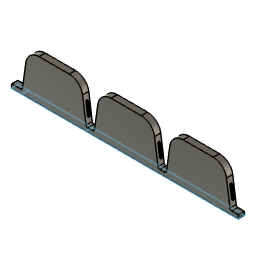
Drawer Organizer v13 (Autodesk Fusion 360 design; units mm, degrees)
Autodesk Fusion 360 part; units mm, degrees
sketch "Schizzo1" plane through (0, 0, 0) normal (0, 0, 1) x (1, 0, 0)
  line L0 (-97, 20) -> (158, 20)
  line L1 (158, 20) -> (158, 13)
  line L2 (158, 13) -> (-97, 13)
  line L3 (-97, 13) -> (-97, 20)
  line L4 (-85, 20) -> (-85, 13)
  line L5 (-13, 20) -> (-13, 13)
  dimension "d1" = 255
  dimension "d2" = 7
  dimension "d3" = 12
  dimension "d4" = 72
  constraint horizontal L0
  constraint vertical L1
  constraint horizontal L2
  constraint vertical L3
  constraint coincident L0 L4.start
  constraint coincident L2 L4.end
  constraint perpendicular L2 L4
  constraint coincident L0 L5.start
  constraint coincident L2 L5.end
  constraint perpendicular L2 L5
  measures "d1" distance of L0.start L0.end
  measures "d2" distance of L0.start L2.end
  measures "d3" distance of L3 L4
  measures "d4" distance of L4 L5
extrude "Estrusione1" add sketch "Schizzo1" along normal blind 4
extrude "Estrusione2" add sketch "Schizzo1" along normal blind 46 contours L0 L2 L4 L5
sketch "Schizzo2" plane through (0, 13, 0) normal (0, -1, 0) x (1, 0, 0)
  line L0 (-85, 4) -> (-97, 4)
  line L1 (-97, 4) -> (-97, 0)
  line L2 (-97, 0) -> (158, 0)
  line L3 (158, 0) -> (158, 4)
  line L4 (158, 4) -> (-13, 4)
  line L5 (-13, 4) -> (-13, 46)
  line L6 (-13, 46) -> (-85, 46)
  line L7 (-85, 46) -> (-85, 4)
  line L8 (-85, 46) -> (-13, 46) construction
  line L9 (-13, 46) -> (-13, 4) construction
  line L10 (-13, 4) -> (-85, 4) construction
  line L11 (-85, 4) -> (-85, 46) construction
  circle A0 centre (-66, 31) radius 15
  line L12 (-49, 46) -> (-49, 4) construction
  circle A1 centre (-32, 31) radius 15
  line L13 (-66, 46) -> (-32, 46)
  line L14 (-85, 4) -> (-80.8499, 33.1166)
  line L15 (-13, 4) -> (-17.1501, 33.1166)
  line L16 (-85, 4) -> (-13, 4)
  line L17 (-66, 46) -> (-85, 46)
  line L18 (-85, 46) -> (-85, 4)
  line L19 (-32, 46) -> (-13, 46)
  line L20 (-13, 46) -> (-13, 4)
  dimension "d9" = 15
  dimension "d10" = 34
  constraint horizontal L8
  constraint vertical L9
  constraint horizontal L10
  constraint vertical L11
  constraint coincident L4.end L5.start
  constraint coincident L6.end L7.start
  constraint tangent L8 A0
  constraint midpoint L8 L12.start
  constraint midpoint L10 L12.end
  constraint symmetric A0 L12 A1
  constraint coincident A0 L13.start
  constraint coincident A1 L13.end
  constraint coincident L8 L13.end
  constraint tangent A1 L13
  constraint coincident L0.start L7.end
  constraint coincident A0 L14.end
  constraint tangent A0 L14
  constraint symmetric L12 L0.start L4.end
  constraint symmetric L12 L14.end L15.end
  constraint perpendicular L11 L17
  constraint symmetric L6.end L12 L5.end
  constraint symmetric L12 L13.start L13.end
  measures "d9" radius of A0
  measures "d10" distance of A0.centre A1.centre
extrude "Estrusione3" cut sketch "Schizzo2" against normal blind 10 contours L6 L7 A0 L14 L17 L18 | L5 L6 A1 L15 L19 L20
pattern_linear "Serie R1" count 3 spacing 81 along (1, 0, 0) of "Estrusione2"
pattern_linear "Serie R2" count 3 spacing 81 along (1, 0, 0) of "Estrusione3"
sketch "Schizzo3" plane through (-83.8663, 0, 11.9537) normal (-0.989994, 0, 0.141107) x (0, -1, 0)
  line L0 (-20, 21.3768) -> (-20, -8.0341)
  line L1 (-20, -8.0341) -> (-13, -8.0341)
  line L2 (-13, -8.0341) -> (-13, 21.3768)
  line L3 (-13, 21.3768) -> (-20, 21.3768)
  line L4 (-20, 21.3768) -> (-13, 21.3768) construction
  line L5 (-13, 21.3768) -> (-13, -8.0341) construction
  line L6 (-13, -8.0341) -> (-20, -8.0341) construction
  line L7 (-20, -8.0341) -> (-20, 21.3768) construction
  line L8 (-16.5, 21.3768) -> (-16.5, -8.0341) construction
  line L9 (-15.8, -0.0341) -> (-17.2, -0.0341)
  line L10 (-17.2, -0.0341) -> (-17.2, 14.9659)
  line L11 (-17.2, 14.9659) -> (-15.8, 14.9659)
  line L12 (-15.8, 14.9659) -> (-15.8, -0.0341)
  line L13 (-15.8, -0.0341) -> (-17.2, 14.9659) construction
  line L14 (-17.2, -0.0341) -> (-15.8, 14.9659) construction
  point P0 (-16.5, 7.4659)
  dimension "d21" = 1.4
  dimension "d22" = 15
  dimension "d23" = 8
  constraint horizontal L4
  constraint vertical L5
  constraint horizontal L6
  constraint vertical L7
  constraint coincident L0.start L3.end
  constraint coincident L1.end L2.start
  constraint midpoint L4 L8.start
  constraint midpoint L6 L8.end
  constraint horizontal L9
  constraint perpendicular L9 L10
  constraint parallel L9 L11
  constraint parallel L10 L12
  constraint coincident L13 P0
  constraint coincident L14 P0
  constraint coincident L8 P0
  measures "d21" distance of L10.end L11.end
  measures "d22" distance of L9.end L10.end
  measures "d23" distance of L6 L9
extrude "Estrusione4" add sketch "Schizzo3" along normal blind 1.5 contours L9 L10 L11 L12
pattern_linear "Serie R3" count 3 spacing 81 along (1, 0, 0) of "Estrusione4"
sketch "Schizzo4" plane through (146.592, 0, 20.8942) normal (0.989994, 0, 0.141107) x (0, 1, 0)
  line L0 (20, -17.065) -> (20, 12.3459)
  line L1 (20, 12.3459) -> (13, 12.3459)
  line L2 (13, 12.3459) -> (13, -17.065)
  line L3 (13, 12.3459) -> (20, 12.3459) construction
  line L4 (20, 12.3459) -> (20, -17.065) construction
  line L5 (20, -17.065) -> (13, -17.065) construction
  line L6 (13, -17.065) -> (13, 12.3459) construction
  line L7 (16.5, 12.3459) -> (16.5, -17.065) construction
  line L8 (17.2, -9.065) -> (15.8, -9.065)
  line L9 (15.8, -9.065) -> (15.8, 5.935)
  line L10 (15.8, 5.935) -> (17.2, 5.935)
  line L11 (17.2, 5.935) -> (17.2, -9.065)
  line L12 (17.2, -9.065) -> (15.8, 5.935) construction
  line L13 (15.8, -9.065) -> (17.2, 5.935) construction
  line L14 (13, -17.065) -> (20, -17.065)
  point P0 (16.5, -1.565)
  dimension "d30" = 1.4
  dimension "d31" = 15
  dimension "d32" = 8
  constraint horizontal L3
  constraint vertical L4
  constraint horizontal L5
  constraint vertical L6
  constraint coincident L1.end L2.start
  constraint coincident L0.start L4.end
  constraint midpoint L3 L7.start
  constraint midpoint L5 L7.end
  constraint horizontal L8
  constraint perpendicular L8 L9
  constraint parallel L8 L10
  constraint parallel L9 L11
  constraint coincident L12 P0
  constraint coincident L13 P0
  constraint coincident L7 P0
  measures "d30" distance of L9.end L10.end
  measures "d31" distance of L8.end L9.end
  measures "d32" distance of L5 L8
extrude "Estrusione5" add sketch "Schizzo4" along normal blind 1.5 contours L8 L9 L10 L11
pattern_linear "Serie R4" count 3 spacing 81 along (-1, 0, 0) of "Estrusione5"
sketch "Schizzo5" plane through (158, 0, 0) normal (1, 0, 0) x (0, 1, 0)
  line L0 (13, 0) -> (20, 0)
  line L1 (20, 0) -> (20, 4)
  line L2 (20, 4) -> (13, 4)
  line L3 (13, 4) -> (13, 0)
  line L4 (13, 4) -> (20, 4) construction
  line L5 (20, 4) -> (20, 0) construction
  line L6 (20, 0) -> (13, 0) construction
  line L7 (13, 0) -> (13, 4) construction
  line L8 (16.5, 4) -> (16.5, 0) construction
  line L9 (13, 2) -> (20, 2) construction
  circle A0 centre (14.5, 2) radius 0.3
  circle A1 centre (18.5, 2) radius 0.3
  circle A2 centre (16.5, 3) radius 0.3
  circle A3 centre (16.5, 1) radius 0.3
  dimension "d39" = 0.6
  dimension "d40" = 0.6
  dimension "d41" = 4
  dimension "d42" = 2
  constraint horizontal L4
  constraint vertical L5
  constraint horizontal L6
  constraint vertical L7
  constraint coincident L2.end L3.start
  constraint coincident L0.end L1.start
  constraint midpoint L4 L8.start
  constraint midpoint L6 L8.end
  constraint midpoint L7 L9.start
  constraint midpoint L5 L9.end
  constraint coincident L9 A0.centre
  constraint symmetric L8 A0 A1
  constraint coincident L8 A2.centre
  constraint symmetric L9 A2 A3
  measures "d39" diameter of A0
  measures "d40" diameter of A2
  measures "d41" distance of A0.centre A1.centre
  measures "d42" distance of A2.centre A3.centre
extrude "Estrusione6" cut sketch "Schizzo5" against normal blind 260 contours A0 | A1 | A2 | A3
fillet "Raccordo1" radius 2 6 edges at (-13, 16.5, 4) (-4, 16.5, 4) (-85, 16.5, 4) (68, 16.5, 4) (77, 16.5, 4) (149, 16.5, 4)
equation "d7 = 42 mm + 4 mm"
equation "d15 = -Spacing"
equation "d19 = Spacing"
equation "d28 = Spacing"
equation "d37 = -Spacing"
equation "d40 = d39"
equation "Spacing = 81 mm" comment "Spacing between blocks"
